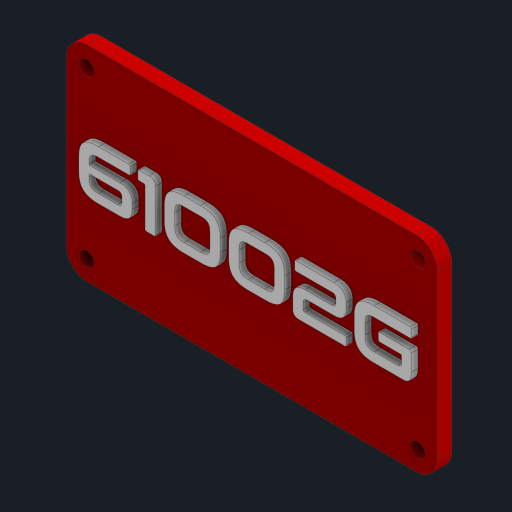
# Autodesk Inventor part: plates
Saved by Autodesk Inventor 2023 (Build 270158000, 158)
## iProperties
Created: 2023-05-25
Part Number: plates
Material: Generic
Document SubType Name: Modeling
Designer: reima
Density: 1 g/cm^3
Appearance: Default
Author: reima
Autodesk Inventor part; units mm, degrees
ref_plane "YZ Plane" through (0, 0, 0) normal (1, 0, 0) x (0, 1, 0)
ref_plane "XZ Plane" through (0, 0, 0) normal (0, 1, 0) x (-1, 0, 0)
ref_plane "XY Plane" through (0, 0, 0) normal (0, 0, 1) x (1, 0, 0)
sketch "Sketch1" plane through (0, 0, 0) normal (0, 0, 1) x (1, 0, 0)
  line L0 (-8.9283, 5.4055) -> (92.1637, 5.4055)
  line L1 (98.5137, -0.9445) -> (98.5137, -51.2365)
  line L2 (92.1637, -57.5865) -> (-8.9283, -57.5865)
  line L3 (-15.2783, -51.2365) -> (-15.2783, -0.9445)
  arc A0 (-8.9283, 5.4055) -> (-15.2783, -0.9445) centre (-8.9283, -0.9445) ccw
  arc A1 (-15.2783, -51.2365) -> (-8.9283, -57.5865) centre (-8.9283, -51.2365) ccw
  arc A2 (92.1637, -57.5865) -> (98.5137, -51.2365) centre (92.1637, -51.2365) ccw
  arc A3 (98.5137, -0.9445) -> (92.1637, 5.4055) centre (92.1637, -0.9445) ccw
  line L4 (-10.8333, -17.9625) -> (89.6237, -17.9625) construction
  line L5 (89.6237, -17.9625) -> (89.6237, -44.7524) construction
  line L6 (89.6237, -44.7524) -> (-10.8333, -44.7524) construction
  line L7 (-10.8333, -44.7524) -> (-10.8333, -17.9625) construction
  line L8 (39.3317, 5.4055) -> (39.3317, -57.5865) construction
  circle A4 centre (-9.1823, -0.9445) radius 2.3368
  circle A5 centre (-9.1823, -51.7445) radius 2.3368
  circle A6 centre (92.6717, -0.9445) radius 2.3368
  circle A7 centre (92.4177, -51.7445) radius 2.3368
  spline S0 degree 2 poles (-3.4722, -17.9625) (-5.6691, -17.9498) (-8.3585, -19.0988) (-9.5833, -21.6241) (-9.5707, -23.7074) knots 0 0 0 1 2 3 3 3
  line L9 (-9.5707, -23.7074) -> (-9.5707, -27.4575)
  spline S1 degree 2 poles (-9.5707, -27.4575) (-9.5833, -29.5408) (-8.3585, -32.0661) (-5.6691, -33.2151) (-3.4722, -33.2025) knots 0 0 0 1 2 3 3 3
  line L10 (-3.4722, -33.2025) -> (2.8915, -33.2025)
  spline S2 degree 2 poles (2.8915, -33.2025) (5.0128, -33.1898) (6.8688, -31.2706) (6.8436, -29.5282) knots 0 0 0 1 2 2 2
  line L11 (6.8436, -29.5282) -> (6.8436, -27.9373)
  spline S3 degree 2 poles (6.8436, -27.9373) (6.8688, -26.1696) (5.1138, -24.263) (3.043, -24.2504) knots 0 0 0 1 2 2 2
  line L12 (3.043, -24.2504) -> (-6.351, -24.2504)
  line L13 (-6.351, -24.2504) -> (-6.351, -23.8337)
  spline S4 degree 2 poles (-6.351, -23.8337) (-6.3762, -22.1418) (-5.1262, -20.8286) (-3.4722, -20.8539) knots 0 0 0 1 2 2 2
  line L14 (-3.4722, -20.8539) -> (5.783, -20.8539)
  spline S5 degree 2 poles (5.783, -20.8539) (6.0229, -20.8539) (6.2628, -20.614) (6.2501, -20.3741) knots 0 0 0 1 2 2 2
  line L15 (6.2501, -20.3741) -> (6.2501, -18.4423)
  spline S6 degree 2 poles (6.2501, -18.4423) (6.2628, -18.2024) (6.0229, -17.9625) (5.783, -17.9625) knots 0 0 0 1 2 2 2
  line L16 (5.783, -17.9625) -> (-3.4722, -17.9625)
  spline S7 degree 2 poles (2.3865, -26.6494) (3.0683, -26.6494) (3.6617, -27.2681) (3.6491, -27.9373) knots 0 0 0 1 2 2 2
  line L17 (3.6491, -27.9373) -> (3.6491, -29.0863)
  spline S8 degree 2 poles (3.6491, -29.0863) (3.6491, -29.7555) (3.043, -30.3994) (2.3612, -30.3994) knots 0 0 0 1 2 2 2
  line L18 (2.3612, -30.3994) -> (-3.4722, -30.3994)
  spline S9 degree 2 poles (-3.4722, -30.3994) (-5.1262, -30.4247) (-6.3762, -29.1241) (-6.351, -27.4322) knots 0 0 0 1 2 2 2
  line L19 (-6.351, -27.4322) -> (-6.351, -26.6494)
  line L20 (-6.351, -26.6494) -> (2.3865, -26.6494)
  spline S10 degree 2 poles (9.0658, -17.9625) (8.8133, -17.9625) (8.5608, -18.2024) (8.5608, -18.4423) knots 0 0 0 1 2 2 2
  line L21 (8.5608, -18.4423) -> (8.5608, -20.3741)
  spline S11 degree 2 poles (8.5608, -20.3741) (8.5608, -20.614) (8.8133, -20.8539) (9.0658, -20.8539) knots 0 0 0 1 2 2 2
  line L22 (9.0658, -20.8539) -> (10.3032, -20.8539)
  spline S12 degree 2 poles (10.3032, -20.8539) (10.5431, -20.8539) (10.7577, -21.0812) (10.7577, -21.3084) knots 0 0 0 1 2 2 2
  line L23 (10.7577, -21.3084) -> (10.7577, -32.7227)
  spline S13 degree 2 poles (10.7577, -32.7227) (10.7577, -32.9626) (10.9976, -33.2025) (11.2375, -33.2025) knots 0 0 0 1 2 2 2
  line L24 (11.2375, -33.2025) -> (13.4724, -33.2025)
  spline S14 degree 2 poles (13.4724, -33.2025) (13.7123, -33.2025) (13.9522, -32.9626) (13.9522, -32.7227) knots 0 0 0 1 2 2 2
  line L25 (13.9522, -32.7227) -> (13.9522, -19.8059)
  spline S15 degree 2 poles (13.9522, -19.8059) (13.9648, -18.8716) (13.0179, -17.9625) (11.9572, -17.9625) knots 0 0 0 1 2 2 2
  line L26 (11.9572, -17.9625) -> (9.0658, -17.9625)
  spline S16 degree 2 poles (22.778, -17.9625) (20.581, -17.9498) (17.8916, -19.0988) (16.6669, -21.6241) (16.6795, -23.7074) knots 0 0 0 1 2 3 3 3
  line L27 (16.6795, -23.7074) -> (16.6795, -27.4575)
  spline S17 degree 2 poles (16.6795, -27.4575) (16.6669, -29.5408) (17.8916, -32.0661) (20.581, -33.2151) (22.778, -33.2025) knots 0 0 0 1 2 3 3 3
  line L28 (22.778, -33.2025) -> (27.8033, -33.2025)
  spline S18 degree 2 poles (27.8033, -33.2025) (30.0003, -33.2151) (32.6897, -32.0661) (33.9145, -29.5408) (33.9018, -27.4575) knots 0 0 0 1 2 3 3 3
  line L29 (33.9018, -27.4575) -> (33.9018, -23.7074)
  spline S19 degree 2 poles (33.9018, -23.7074) (33.9145, -21.6241) (32.6897, -19.0988) (30.0003, -17.9498) (27.8033, -17.9625) knots 0 0 0 1 2 3 3 3
  line L30 (27.8033, -17.9625) -> (22.778, -17.9625)
  spline S20 degree 2 poles (19.8992, -23.8337) (19.874, -22.1418) (21.124, -20.8286) (22.778, -20.8539) knots 0 0 0 1 2 2 2
  line L31 (22.778, -20.8539) -> (27.8033, -20.8539)
  spline S21 degree 2 poles (27.8033, -20.8539) (29.4574, -20.8286) (30.7074, -22.1418) (30.6821, -23.8337) knots 0 0 0 1 2 2 2
  line L32 (30.6821, -23.8337) -> (30.6821, -27.3312)
  spline S22 degree 2 poles (30.6821, -27.3312) (30.7074, -29.0231) (29.4574, -30.3363) (27.8033, -30.311) knots 0 0 0 1 2 2 2
  line L33 (27.8033, -30.311) -> (22.778, -30.311)
  spline S23 degree 2 poles (22.778, -30.311) (21.124, -30.3363) (19.874, -29.0231) (19.8992, -27.3312) knots 0 0 0 1 2 2 2
  line L34 (19.8992, -27.3312) -> (19.8992, -23.8337)
  spline S24 degree 2 poles (42.5256, -17.9625) (40.3286, -17.9498) (37.6392, -19.0988) (36.4145, -21.6241) (36.4271, -23.7074) knots 0 0 0 1 2 3 3 3
  line L35 (36.4271, -23.7074) -> (36.4271, -27.4575)
  spline S25 degree 2 poles (36.4271, -27.4575) (36.4145, -29.5408) (37.6392, -32.0661) (40.3286, -33.2151) (42.5256, -33.2025) knots 0 0 0 1 2 3 3 3
  line L36 (42.5256, -33.2025) -> (47.5509, -33.2025)
  spline S26 degree 2 poles (47.5509, -33.2025) (49.7479, -33.2151) (52.4373, -32.0661) (53.6621, -29.5408) (53.6494, -27.4575) knots 0 0 0 1 2 3 3 3
  line L37 (53.6494, -27.4575) -> (53.6494, -23.7074)
  spline S27 degree 2 poles (53.6494, -23.7074) (53.6621, -21.6241) (52.4373, -19.0988) (49.7479, -17.9498) (47.5509, -17.9625) knots 0 0 0 1 2 3 3 3
  line L38 (47.5509, -17.9625) -> (42.5256, -17.9625)
  spline S28 degree 2 poles (39.6468, -23.8337) (39.6216, -22.1418) (40.8716, -20.8286) (42.5256, -20.8539) knots 0 0 0 1 2 2 2
  line L39 (42.5256, -20.8539) -> (47.5509, -20.8539)
  spline S29 degree 2 poles (47.5509, -20.8539) (49.205, -20.8286) (50.455, -22.1418) (50.4297, -23.8337) knots 0 0 0 1 2 2 2
  line L40 (50.4297, -23.8337) -> (50.4297, -27.3312)
  spline S30 degree 2 poles (50.4297, -27.3312) (50.455, -29.0231) (49.205, -30.3363) (47.5509, -30.311) knots 0 0 0 1 2 2 2
  line L41 (47.5509, -30.311) -> (42.5256, -30.311)
  spline S31 degree 2 poles (42.5256, -30.311) (40.8716, -30.3363) (39.6216, -29.0231) (39.6468, -27.3312) knots 0 0 0 1 2 2 2
  line L42 (39.6468, -27.3312) -> (39.6468, -23.8337)
  spline S32 degree 2 poles (57.1596, -17.9625) (56.907, -17.9625) (56.6798, -18.2024) (56.6798, -18.4423) knots 0 0 0 1 2 2 2
  line L43 (56.6798, -18.4423) -> (56.6798, -20.3741)
  spline S33 degree 2 poles (56.6798, -20.3741) (56.6798, -20.614) (56.907, -20.8539) (57.1596, -20.8539) knots 0 0 0 1 2 2 2
  line L44 (57.1596, -20.8539) -> (68.1697, -20.8539)
  spline S34 degree 2 poles (68.1697, -20.8539) (68.7758, -20.8539) (69.3187, -21.5231) (69.3187, -22.1039) knots 0 0 0 1 2 2 2
  line L45 (69.3187, -22.1039) -> (69.3187, -23.0382)
  spline S35 degree 2 poles (69.3187, -23.0382) (69.3187, -23.6443) (68.7758, -24.263) (68.1824, -24.263) knots 0 0 0 1 2 2 2
  line L46 (68.1824, -24.263) -> (59.9121, -24.263)
  spline S36 degree 2 poles (59.9121, -24.263) (58.0434, -24.2756) (56.1116, -26.1948) (56.1116, -28.0004) knots 0 0 0 1 2 2 2
  line L47 (56.1116, -28.0004) -> (56.1116, -31.359)
  spline S37 degree 2 poles (56.1116, -31.359) (56.099, -32.2934) (57.0459, -33.2025) (58.1318, -33.2025) knots 0 0 0 1 2 2 2
  line L48 (58.1318, -33.2025) -> (72.0208, -33.2025)
  spline S38 degree 2 poles (72.0208, -33.2025) (72.2607, -33.2025) (72.5132, -32.9626) (72.5132, -32.7227) knots 0 0 0 1 2 2 2
  line L49 (72.5132, -32.7227) -> (72.5132, -30.7908)
  spline S39 degree 2 poles (72.5132, -30.7908) (72.5132, -30.5509) (72.2607, -30.311) (72.0208, -30.311) knots 0 0 0 1 2 2 2
  line L50 (72.0208, -30.311) -> (59.7606, -30.311)
  spline S40 degree 2 poles (59.7606, -30.311) (59.5333, -30.311) (59.3313, -30.0837) (59.3313, -29.8565) knots 0 0 0 1 2 2 2
  line L51 (59.3313, -29.8565) -> (59.3313, -28.0004)
  spline S41 degree 2 poles (59.3313, -28.0004) (59.3313, -27.3817) (59.8742, -26.763) (60.4677, -26.763) knots 0 0 0 1 2 2 2
  line L52 (60.4677, -26.763) -> (68.7379, -26.763)
  spline S42 degree 2 poles (68.7379, -26.763) (70.6066, -26.7504) (72.5385, -24.8312) (72.5385, -23.0382) knots 0 0 0 1 2 2 2
  line L53 (72.5385, -23.0382) -> (72.5385, -21.5105)
  spline S43 degree 2 poles (72.5385, -21.5105) (72.5385, -19.9069) (70.6571, -17.9877) (68.6874, -17.9625) knots 0 0 0 1 2 2 2
  line L54 (68.6874, -17.9625) -> (57.1596, -17.9625)
  spline S44 degree 2 poles (81.0612, -17.9625) (78.8643, -17.9498) (76.1748, -19.0988) (74.9501, -21.6367) (74.9627, -23.7201) knots 0 0 0 1 2 3 3 3
  line L55 (74.9627, -23.7201) -> (74.9627, -27.4575)
  spline S45 degree 2 poles (74.9627, -27.4575) (74.9501, -29.5408) (76.1748, -32.0661) (78.8643, -33.2151) (81.0612, -33.2025) knots 0 0 0 1 2 3 3 3
  line L56 (81.0612, -33.2025) -> (89.8492, -33.2025)
  spline S46 degree 2 poles (89.8492, -33.2025) (91.1623, -33.2277) (92.5386, -31.6873) (92.5512, -29.8817) knots 0 0 0 1 2 2 2
  line L57 (92.5512, -29.8817) -> (92.5512, -24.8059)
  spline S47 degree 2 poles (92.5512, -24.8059) (92.5512, -24.1494) (91.8946, -24.1494) knots 0 0 0 1 1 1
  line L58 (91.8946, -24.1494) -> (82.8163, -24.1494)
  spline S48 degree 2 poles (82.8163, -24.1494) (82.589, -24.1494) (82.3491, -24.4019) (82.3365, -24.6544) knots 0 0 0 1 2 2 2
  line L59 (82.3365, -24.6544) -> (82.3365, -26.2832)
  spline S49 degree 2 poles (82.3365, -26.2832) (82.3491, -26.5357) (82.589, -26.7883) (82.8163, -26.7883) knots 0 0 0 1 2 2 2
  line L60 (82.8163, -26.7883) -> (89.1926, -26.7883)
  spline S50 degree 2 poles (89.1926, -26.7883) (89.3441, -26.7883) (89.4578, -26.9272) (89.4578, -27.0661) knots 0 0 0 1 2 2 2
  line L61 (89.4578, -27.0661) -> (89.4578, -28.8337)
  spline S51 degree 2 poles (89.4578, -28.8337) (89.4578, -29.5534) (88.9401, -30.1721) (88.3719, -30.1595) knots 0 0 0 1 2 2 2
  line L62 (88.3719, -30.1595) -> (81.1875, -30.1595)
  spline S52 degree 2 poles (81.1875, -30.1595) (79.5335, -30.1848) (78.2708, -28.8842) (78.2961, -27.1797) knots 0 0 0 1 2 2 2
  line L63 (78.2961, -27.1797) -> (78.2961, -24.0484)
  spline S53 degree 2 poles (78.2961, -24.0484) (78.2708, -22.3438) (79.5335, -21.0433) (81.1875, -21.0812) knots 0 0 0 1 2 2 2
  line L64 (81.1875, -21.0812) -> (92.0967, -21.0812)
  spline S54 degree 2 poles (92.0967, -21.0812) (92.3366, -21.0812) (92.5765, -20.8286) (92.5765, -20.5761) knots 0 0 0 1 2 2 2
  line L65 (92.5765, -20.5761) -> (92.5765, -18.4423)
  spline S55 degree 2 poles (92.5765, -18.4423) (92.5765, -18.2024) (92.3366, -17.9625) (92.0967, -17.9625) knots 0 0 0 1 2 2 2
  line L66 (92.0967, -17.9625) -> (81.0612, -17.9625)
  point P0 (0, 0)
  point P1 (98.5137, -57.5865)
  point P2 (98.5137, 5.4055)
  point P3 (-15.2783, -57.5865)
  dimension "d0" = 113.792
  dimension "d1" = 62.992
  dimension "d2" = 6.35
  dimension "d3" = 23.368
  dimension "d4" = 8.89
  dimension "d5" = 4.445
  dimension "d6" = 4.6736
  dimension "d7" = 4.6736
  dimension "d8" = 50.8
  dimension "d9" = 6.096
  dimension "d10" = 6.35
  dimension "d11" = 4.6736
  dimension "d12" = 4.6736
  dimension "d13" = 101.6
  dimension "d14" = 6.096
  dimension "d15" = 101.6
  dimension "d16" = 50.8
  dimension "d17" = 6.35
  constraints: 10 end point, 8 centre point, 8 point on circle, 8 point on line, 8 tangent, 3 equal radius, 2 parallel, 2 perpendicular, 1 horizontal, 2 other
  measures "d0" distance of point (98.514, -57.586) point (-15.278, -57.586)
  measures "d1" distance of point (98.514, 5.406) point (98.514, -57.586)
  measures "d2" radius of A0
  measures "d3" distance between parallel lines of L0 L4
  measures "d4" distance between parallel lines of L1 L5
  measures "d5" distance between parallel lines of L3 L7
  measures "d6" diameter of A4
  measures "d7" diameter of A5
  measures "d8" distance of A5.centre A4.centre
  measures "d9" distance from line of L3 A5.centre
  measures "d10" distance from line of L0 A4.centre
  measures "d11" diameter of A6
  measures "d12" diameter of A7
  measures "d13" distance of A0.centre A6.centre
  measures "d14" distance from line of L3 A4.centre
  measures "d15" distance of A5.centre A7.centre
  measures "d16" vertical distance of A7.centre A6.centre
  measures "d17" distance from line of L0 A6.centre
extrude "Extrusion1" add sketch "Sketch1" along normal blind 4.445 contours L0 A3 L1 A2 L2 A1 L3 A0 | L16 S6 L15 S5 L14 S4 L13 L12 S3 L11 S2 L10 S1 L9 S0 | S7 L17 S8 L18 S9 L19 L20 | L26 S15 L25 S14 L24 S13 L23 S12 L22 S11 L21 S10 | L30 S19 L29 S18 L28 S17 L27 S16 | S20 L31 S21 L32 S22 L33 S23 L34 | L38 S27 L37 S26 L36 S25 L35 S24 | S28 L39 S29 L40 S30 L41 S31 L42 | L54 S43 L53 S42 L52 S41 L51 S40 L50 S39 L49 S38 L48 S37 L47 S36 L46 S35 L45 S34 L44 S33 L43 S32 | L66 S55 L65 S54 L64 S53 L63 S52 L62 S51 L61 S50 L60 S49 L59 S48 L58 S47 L57 S46 L56 S45 L55 S44
extrude "Extrusion2" add sketch "Sketch1" along normal blind 6.35 contours L16 S6 L15 S5 L14 S4 L13 L12 S3 L11 S2 L10 S1 L9 S0 | L26 S15 L25 S14 L24 S13 L23 S12 L22 S11 L21 S10 | L30 S19 L29 S18 L28 S17 L27 S16 | L38 S27 L37 S26 L36 S25 L35 S24 | L54 S43 L53 S42 L52 S41 L51 S40 L50 S39 L49 S38 L48 S37 L47 S36 L46 S35 L45 S34 L44 S33 L43 S32 | L66 S55 L65 S54 L64 S53 L63 S52 L62 S51 L61 S50 L60 S49 L59 S48 L58 S47 L57 S46 L56 S45 L55 S44
body "Solid1"
